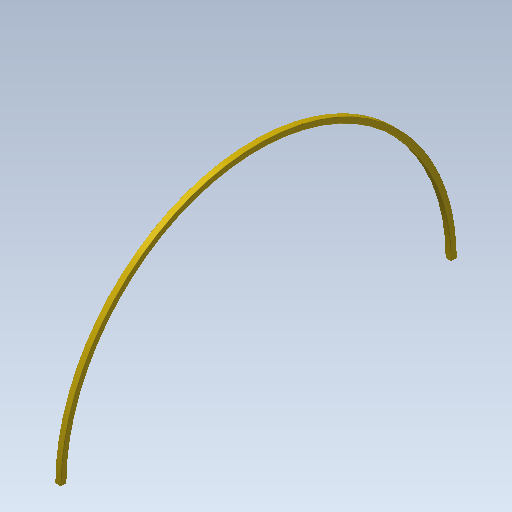
# Autodesk Inventor part: Luk R2000
Saved by Autodesk Inventor 2021 (Build 250183000, 183)
## iProperties
Created: 2024-04-08
Part Number: Luk R2000
Material: Steel
Document SubType Name: Modeling
Designer: Michal
Density: 7.85 g/cm^3
Appearance: Glossy - Gold
Author: Michal
Autodesk Inventor part; units mm, degrees
ref_plane "YZ Plane" through (0, 0, 0) normal (1, 0, 0) x (0, 1, 0)
ref_plane "XZ Plane" through (0, 0, 0) normal (0, 1, 0) x (-1, 0, 0)
ref_plane "XY Plane" through (0, 0, 0) normal (0, 0, 1) x (1, 0, 0)
sketch "Sketch1" plane through (0, 0, 0) normal (0, 1, 0) x (-1, 0, 0)
  line L0 (-12, 14) -> (12, 14) construction
  line L1 (14, 12) -> (14, -12) construction
  line L2 (12, -14) -> (-12, -14) construction
  line L3 (-14, -12) -> (-14, 12) construction
  line L4 (-14, 14) -> (14, -14) construction
  line L5 (14, 14) -> (-14, -14) construction
  arc A0 (14, 12) -> (12, 14) centre (12, 12) ccw construction
  arc A1 (12, -14) -> (14, -12) centre (12, -12) ccw construction
  arc A2 (-14, -12) -> (-12, -14) centre (-12, -12) ccw construction
  arc A3 (-12, 14) -> (-14, 12) centre (-12, 12) ccw construction
  line L6 (-12, -15) -> (12, -15)
  arc A4 (12, -15) -> (15, -12) centre (12, -12) ccw
  line L7 (15, -12) -> (15, 12)
  arc A5 (15, 12) -> (12, 15) centre (12, 12) ccw
  line L8 (12, 15) -> (-12, 15)
  arc A6 (-12, 15) -> (-15, 12) centre (-12, 12) ccw
  line L9 (-15, 12) -> (-15, -12)
  arc A7 (-15, -12) -> (-12, -15) centre (-12, -12) ccw
  line L10 (13, -12) -> (13, 12)
  arc A8 (13, 12) -> (12, 13) centre (12, 12) ccw
  line L11 (12, 13) -> (-12, 13)
  arc A9 (-12, 13) -> (-13, 12) centre (-12, 12) ccw
  line L12 (-13, 12) -> (-13, -12)
  arc A10 (-13, -12) -> (-12, -13) centre (-12, -12) ccw
  line L13 (-12, -13) -> (12, -13)
  arc A11 (12, -13) -> (13, -12) centre (12, -12) ccw
  point P0 (0, 0)
  point P1 (0, 0)
  point P2 (0, 0)
  dimension "d10" = 2
  dimension "depth" = 30
  dimension "width" = 30
  dimension "thickness" = 2
  constraints: 28 end point, 24 point on circle, 12 centre point, 8 point on line, 8 tangent, 6 parallel, 3 equal radius, 3 midpoint, 3 perpendicular, 1 coincident, 1 horizontal, 15 other
  measures "d10" radius of A0
  measures "depth" distance between parallel lines of L6 L8
  measures "width" distance between parallel lines of L9 L7
  measures "thickness" distance between parallel lines of L10 L7
sketch "Sketch3" plane through (0, 0, 0) normal (1, 0, 0) x (0, 1, 0)
  line L0 (0, 0) -> (0, 2000) construction
  arc A0 (0, 0) -> (0, 2000) centre (0, 1000) ccw
  line L1 (0, -400) -> (0, 2400) projected
  line L2 (-200, 0) -> (1200, 0) projected
  dimension "d30" = 2000
  dimension "d31" = 1000
  constraints: 2 end point, 2 point on circle, 2 point on line, 1 centre point, 1 collinear
  measures "d30" distance of L0.start L0.end
  measures "d31" radius of A0
sweep "Sweep1" add profiles "Sketch1" path "Sketch3" path curves A0
sketch "Sketch5" plane through (-15, 0, 1000) normal (-1, 0, 0) x (0, 0, 1)
  arc A0 (1000, 0) -> (-1000, 0) centre (0, 0) ccw construction
  line L0 (-1012, 0) -> (-988, 0) projected
  line L1 (1012, 0) -> (988, 0) projected
  point P0 (-1000, 0)
  point P1 (-998.7492, 50)
  point P2 (-995.0016, 99.8594)
  point P3 (1000, 0)
  point P4 (998.7492, 50)
  point P5 (995.0016, 99.8594)
  dimension "d46" = 50
  dimension "d51" = 50
  dimension "d52" = 50
  dimension "d53" = 50
  constraints: 7 other
  measures "d46" distance from line of L0 point (-998.749, 50)
  measures "d51" distance of point (998.749, 50) point (995.002, 99.859)
  measures "d52" distance from line of point (998.749, 50) L1
  measures "d53" distance of point (-995.002, 99.859) point (-998.749, 50)
hole "Hole3" at (-15, 50, 1.2508) at (-15, 99.8594, 4.9984) at (-15, 50, 1998.7492) at (-15, 99.8594, 1995.0016) direction (1, 0, 0) diameter 9 depth 20.2 tip angle 118
equation "\"d10\" = thickness"
equation "\"d31\" = 0.5 * d30"
body "Solid2"
